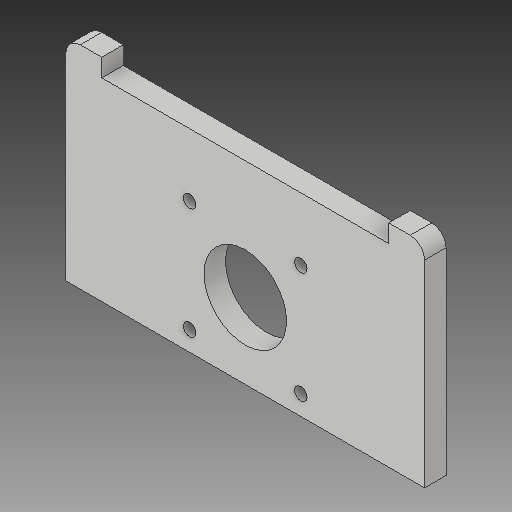
# Autodesk Inventor part: Tope riel motor
Saved by Autodesk Inventor 2019 (Build 230136000, 136)
## iProperties
Created: 2020-02-01
Part Number: Tope riel motor
Material: Generic
Document SubType Name: Modeling
Designer: Elías Sánchez
Density: 1 g/cm^3
Appearance: Default
Description: Corte Láser
Author: Elías Sánchez
Revision Number: IR
Autodesk Inventor part; units mm, degrees
ref_plane "YZ Plane" through (0, 0, 0) normal (1, 0, 0) x (0, 1, 0)
ref_plane "XZ Plane" through (0, 0, 0) normal (0, 1, 0) x (-1, 0, 0)
ref_plane "XY Plane" through (0, 0, 0) normal (0, 0, 1) x (1, 0, 0)
sketch "Sketch1" plane through (0, 0, 0) normal (0, 0, 1) x (1, 0, 0)
  line L0 (-50, 0) -> (50, 0)
  circle A0 centre (-15.5, 36.5) radius 1.75
  circle A1 centre (15.5, 36.5) radius 1.75
  circle A2 centre (-15.5, 5.5) radius 1.75
  circle A3 centre (15.5, 5.5) radius 1.75
  circle A4 centre (0, 21) radius 11.5
  line L1 (-50, 0) -> (-50, 59)
  line L2 (50, 59) -> (50, 0)
  line L3 (-50, 59) -> (-40, 59)
  line L4 (-40, 59) -> (-40, 54)
  line L5 (-40, 54) -> (40, 54)
  line L6 (40, 54) -> (40, 59)
  line L7 (40, 59) -> (50, 59)
  point P0 (0, 0)
  point P1 (0, 42)
  point P2 (0, 0)
  point P3 (0, 54)
  dimension "d4" = 100
  dimension "d13" = 3.5
  dimension "d14" = 3.5
  dimension "d15" = 15.5
  dimension "d16" = 15.5
  dimension "d17" = 36.5
  dimension "d21" = 3.5
  dimension "d22" = 3.5
  dimension "d23" = 31
  dimension "d24" = 23
  dimension "d28" = 21
  dimension "d31" = 80
  dimension "d32" = 5
  dimension "d33" = 59
  dimension "d34" = 54
  constraints: 16 end point, 5 centre point, 5 vertical alignment, 4 perpendicular, 2 coincident, 2 horizontal, 2 horizontal alignment, 2 midpoint, 1 point on line, 1 vertical
  measures "d4" distance of L0.start L0.end
  measures "d13" diameter of A0
  measures "d14" diameter of A1
  measures "d15" horizontal distance of point (0, 0) A0.centre
  measures "d16" horizontal distance of point (0, 0) A1.centre
  measures "d17" distance from line of L0 A1.centre
  measures "d21" diameter of A2
  measures "d22" diameter of A3
  measures "d23" distance of A3.centre A1.centre
  measures "d24" diameter of A4
  measures "d28" distance from line of L0 A4.centre
  measures "d31" distance of L4.end L5.end
  measures "d32" distance of L3.end L4.end
  measures "d33" distance of L2.start L0.end
  measures "d34" distance between parallel lines of L0 L5
extrude "Extrusion2" add sketch "Sketch1" along normal blind 6
fillet "Fillet3" radius 4 2 edges at (-50, 59, 3) (50, 59, 3)
equation "\"d14\" = d13"
equation "\"d16\" = d15"
equation "\"d21\" = d13"
equation "\"d22\" = d13"
body "Solid2"
